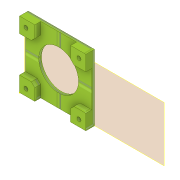
# Autodesk Inventor part: 30_Z_Stage_Adapterplate
Saved by Autodesk Inventor 2019 (Build 230136000, 136)
## iProperties
Created: 2019-06-20
Part Number: 30_Z_Stage_Adapterplate
Material: Generic
Document SubType Name: Modeling
Designer: diederichbenedict
Density: 1 g/cm^3
Appearance: IPHT_GREEN
Author: diederichbenedict
Autodesk Inventor part; units mm, degrees
ref_plane "YZ Plane" through (0, 0, 0) normal (1, 0, 0) x (0, 1, 0)
ref_plane "XZ Plane" through (0, 0, 0) normal (0, 1, 0) x (-1, 0, 0)
ref_plane "XY Plane" through (0, 0, 0) normal (0, 0, 1) x (1, 0, 0)
ref_plane "Work Plane1" through (0, 0, 0) normal (0, 0, 1) x (1, 0, 0)
sketch "Sketch1" plane through (0, 0, 0) normal (0, 0, 1) x (1, 0, 0)
  circle A0 centre (44.9, 44.85) radius 3.1 construction
  arc A1 (2, 43.7546) -> (2, 45.9454) centre (4.9, 44.85) ccw construction
  line L0 (2, 39.7) -> (2, 43.7546) construction
  line L1 (97.8, 39.7) -> (2, 39.7) construction
  line L2 (97.8, 43.9046) -> (97.8, 39.7) construction
  arc A2 (94.119, 48) -> (97.8, 43.9046) centre (94.9, 45) ccw construction
  line L3 (55.681, 48) -> (94.119, 48) construction
  arc A3 (54.119, 48) -> (55.681, 48) centre (54.9, 45) ccw construction
  line L4 (29.1188, 48) -> (54.119, 48) construction
  line L5 (2, 45.9454) -> (2, 48) construction
  arc A4 (4.9, 2) -> (2, 5.7681) centre (4.9, 5) ccw construction
  line L6 (44.9, 2) -> (4.9, 2) construction
  circle A5 centre (44.9, 5) radius 3 construction
  line L7 (54.9, 2) -> (44.9, 2) construction
  circle A6 centre (54.9, 5) radius 3 construction
  line L8 (94.9, 2) -> (54.9, 2) construction
  arc A7 (97.8, 5.7681) -> (94.9, 2) centre (94.9, 5) ccw construction
  line L9 (97.8, 39.7) -> (97.8, 5.7681) construction
  line L10 (91.397, 39.7) -> (97.8, 39.7) construction
  line L11 (91.397, 10.3) -> (91.397, 39.7) construction
  line L12 (8.403, 10.3) -> (91.397, 10.3) construction
  line L13 (8.403, 10.3) -> (8.403, 39.7) construction
  line L14 (2, 39.7) -> (8.403, 39.7) construction
  line L15 (2, 5.7681) -> (2, 39.7) construction
  arc A8 (99.8, 48) -> (97.8, 50) centre (97.8, 48) ccw construction
  arc A9 (97.8, 0) -> (99.8, 2) centre (97.8, 2) ccw construction
  arc A10 (2, 50) -> (0, 48) centre (2, 48) ccw construction
  arc A11 (0, 2) -> (2, 0) centre (2, 2) ccw construction
  line L16 (0, 50) -> (99.8, 50)
  line L17 (99.8, 50) -> (99.8, 0)
  line L18 (99.8, 0) -> (0, 0)
  line L19 (0, 0) -> (0, 50)
  circle A12 centre (94.9, 45) radius 1.6 construction
  arc A13 (93.935, 3.8516) -> (95.865, 3.8516) centre (94.9, 5) ccw construction
  circle A14 centre (54.9, 5) radius 1.5 construction
  circle A15 centre (54.9, 45) radius 1.6 construction
  circle A16 centre (44.9, 44.85) radius 1.6 construction
  circle A17 centre (44.9, 5) radius 1.5 construction
  circle A18 centre (4.9, 44.85) radius 1.6 construction
  circle A19 centre (4.9, 5) radius 1.5 construction
  line L20 (0, 50) -> (50, 50) construction
  line L21 (50, 50) -> (50, 0) construction
  line L22 (50, 0) -> (0, 0) construction
  line L23 (0, 0) -> (0, 50) construction
  line L24 (50, 50) -> (0, 50)
  line L25 (0, 50) -> (0, 0)
  line L26 (0, 0) -> (50, 0)
  line L27 (50, 0) -> (50, 50)
  circle A20 centre (25, 25) radius 15
  circle A21 centre (44.9, 44.85) radius 1.5
  circle A22 centre (4.9, 44.85) radius 1.5
  circle A23 centre (4.9, 5) radius 1.5
  circle A24 centre (44.9, 5) radius 1.5
  line L28 (29.1188, 48) -> (29.1188, 47.25) projected
  line L29 (29.1188, 47.25) -> (20.2352, 47.25) projected
  line L30 (20.2352, 47.25) -> (20.2352, 48) projected
  line L31 (2, 48) -> (20.2352, 48) projected
  point P0 (0, 0)
  dimension "d0" = 50
  dimension "d1" = 50
  dimension "d2" = 30
  dimension "d3" = 3
  dimension "d4" = 3
  dimension "d5" = 3
  dimension "d6" = 3
  constraints: 24 end point, 6 parallel, 5 centre point, 4 coincident, 3 horizontal, 3 perpendicular, 2 vertical alignment
  measures "d0" distance of L21.end L22.end
  measures "d1" distance of L20.end L21.end
  measures "d2" diameter of A20
  measures "d3" diameter of A21
  measures "d4" diameter of A22
  measures "d5" diameter of A23
  measures "d6" diameter of A24
extrude "Extrusion1" add sketch "Sketch1" along normal blind 2 contours L16 L27 L18 L19
sketch "Sketch2" plane through (0, 0, 2) normal (0, 0, 1) x (1, 0, 0)
  circle A0 centre (25, 25) radius 15 projected
  circle A1 centre (44.9, 5) radius 1.5 projected
  circle A2 centre (4.9, 5) radius 1.5 projected
  circle A3 centre (4.9, 44.85) radius 1.5 projected
  circle A4 centre (44.9, 44.85) radius 1.5 projected
  line L0 (50, 50) -> (0, 50) projected
  line L1 (0, 50) -> (0, 0) projected
  line L2 (0, 0) -> (50, 0) projected
  line L3 (50, 0) -> (50, 50) projected
  circle A5 centre (25, 25) radius 15 projected
  circle A6 centre (25, 25) radius 21
  point P0 (0, 0)
  dimension "d9" = 42
  constraints: 1 centre point, 1 coincident
  measures "d9" diameter of A6
extrude "Extrusion2" add sketch "Sketch2" along normal blind 4.5 contours L3 L2 L1 L0
sketch "Sketch3" plane through (0, 0, 6.5) normal (0, 0, 1) x (1, 0, 0)
  point P0 (0, 0)
sketch "Sketch4" plane through (0, 0, 6.5) normal (0, 0, 1) x (1, 0, 0)
  arc A0 (5.5835, 17) -> (44.4165, 17) centre (25, 25) ccw construction
  line L0 (0.75, 17) -> (5.5835, 17) construction
  line L1 (0.75, 17) -> (0.75, 33) construction
  line L2 (5.5835, 33) -> (0.75, 33) construction
  arc A1 (44.4165, 33) -> (5.5835, 33) centre (25, 25) ccw construction
  line L3 (49.25, 33) -> (44.4165, 33) construction
  line L4 (49.25, 33) -> (49.25, 17) construction
  line L5 (44.4165, 17) -> (49.25, 17) construction
  line L6 (0, 0) -> (50, 0) projected
  line L7 (38.5, 50) -> (11.5, 50)
  line L8 (11.5, 50) -> (11.5, 0)
  line L9 (11.5, 0) -> (38.5, 0)
  line L10 (38.5, 0) -> (38.5, 50)
  line L11 (38.5, 50) -> (11.5, 0) construction
  line L12 (11.5, 50) -> (38.5, 0) construction
  line L13 (0, 50) -> (0, 0) projected
  line L14 (50, 38.5) -> (0, 38.5)
  line L15 (0, 38.5) -> (0, 11.5)
  line L16 (0, 11.5) -> (50, 11.5)
  line L17 (50, 11.5) -> (50, 38.5)
  line L18 (50, 38.5) -> (0, 11.5) construction
  line L19 (0, 38.5) -> (50, 11.5) construction
  circle A2 centre (4.9, 45) radius 0.6526 projected
  circle A3 centre (44.9, 45) radius 0.6526 projected
  circle A4 centre (4.9, 5) radius 0.6526 projected
  circle A5 centre (44.9, 5) radius 0.6526 projected
  line L20 (0, 0) -> (50, 0) projected
  line L21 (50, 0) -> (50, 50) projected
  line L22 (50, 50) -> (0, 50) projected
  line L23 (0, 50) -> (0, 0) projected
  dimension "d12" = 27
  dimension "d13" = 27
  constraints: 24 end point, 4 midpoint, 4 parallel, 2 horizontal, 2 perpendicular, 2 point on line
  measures "d12" distance of L9.end L8.end
  measures "d13" distance of L15.end L14.end
extrude "Extrusion3" cut sketch "Sketch4" against normal up to surface (4.5 mm away) contours L8 L16 L10 L6 | L13 L14 L8 L16 | L8 L14 L10 L16 | L10 L14 L17 L16 | L8 L7 L10 L14
body "Solid1"
